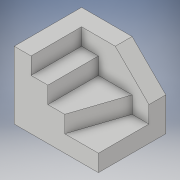
# Autodesk Inventor part: 零件15
Saved by Autodesk Inventor 2019 (Build 230136000, 136)
## iProperties
Created: 2020-09-18
Part Number: 零件15
Material: 一般
Document SubType Name: Modeling
Designer: jay
Density: 1 g/cm^3
Appearance: 預設
Author: jay
Autodesk Inventor part; units mm, degrees
ref_plane "YZ Plane" through (0, 0, 0) normal (1, 0, 0) x (0, 1, 0)
ref_plane "XZ Plane" through (0, 0, 0) normal (0, 1, 0) x (-1, 0, 0)
ref_plane "XY Plane" through (0, 0, 0) normal (0, 0, 1) x (1, 0, 0)
sketch "草圖1" plane through (0, 0, 0) normal (0, 0, 1) x (1, 0, 0)
  line L0 (0, 0) -> (50, 0)
  line L1 (50, 0) -> (50, 20)
  line L2 (50, 20) -> (30, 40)
  line L3 (30, 40) -> (0, 40)
  line L4 (0, 40) -> (0, 0)
  dimension "d0" = 40
  dimension "d1" = 50
  dimension "d2" = 20
  dimension "d3" = 30
  constraints: 10 end point, 2 perpendicular, 1 horizontal, 1 parallel
  measures "d0" distance of L3.end L0.start
  measures "d1" distance of L0.start L0.end
  measures "d2" distance of L0.end L1.end
  measures "d3" distance of L2.end L3.end
extrude "擠出1" add sketch "草圖1" along normal blind 10
sketch "草圖2" plane through (0, 0, 10) normal (0, 0, 1) x (1, 0, 0)
  line L0 (30, 40) -> (0, 40) projected
  line L1 (0, 40) -> (0, 0)
  line L2 (50, 0) -> (50, 20) projected
  line L3 (0, 0) -> (50, 0)
  line L4 (50, 0) -> (50, 10)
  line L5 (50, 10) -> (40, 10)
  line L6 (40, 10) -> (40, 20)
  line L7 (40, 20) -> (20, 20)
  line L8 (20, 20) -> (20, 30)
  line L9 (20, 30) -> (10, 30)
  line L10 (10, 30) -> (10, 40)
  line L11 (10, 40) -> (0, 40)
  dimension "d6" = 10
  dimension "d7" = 10
  dimension "d8" = 10
  dimension "d9" = 10
  dimension "d10" = 20
  constraints: 20 end point, 6 perpendicular, 2 horizontal, 2 vertical, 1 midpoint, 1 point on line
  measures "d6" distance between parallel lines of L1 L10
  measures "d7" distance of L9.end L10.end
  measures "d8" distance of L8.end L9.end
  measures "d9" distance of L5.end L6.end
  measures "d10" distance of L6.end L7.end
extrude "擠出2" add sketch "草圖2" along normal blind 30
chamfer "倒角1" distance 10 distance2 30 1 edges at (40, 15, 40) measured on face at (20, 10, 40)
